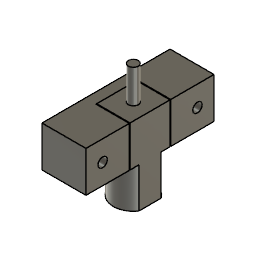
DC Motor (Autodesk Fusion 360 design; units mm, degrees)
Autodesk Fusion 360 part; units mm, degrees
sketch "Çizim1" plane through (0, 0, 0) normal (0, 0, 1) x (1, 0, 0)
  line L0 (5, 6) -> (-5, 6)
  line L1 (-5, 6) -> (-5, -6)
  line L2 (-5, -6) -> (5, -6)
  line L3 (5, -6) -> (5, 6)
  line L4 (5, 6) -> (-5, -6) construction
  line L5 (-5, 6) -> (5, -6) construction
  dimension "d1" = 10
  dimension "d2" = 12
  constraint horizontal L0
  constraint perpendicular L0 L1
  constraint parallel L0 L2
  constraint parallel L1 L3
  constraint coincident L4 origin
  constraint coincident L5 origin
  measures "d1" distance of L1.end L2.end
  measures "d2" distance of L0.end L1.end
extrude "Ekstrüzyon1" add sketch "Çizim1" along normal blind 24.2 makes body 1
sketch "Çizim2" plane through (0, 0, 24.2) normal (0, 0, 1) x (-1, 0, 0)
  line L0 (-5, 6) -> (-5, -6)
  line L1 (-5, -6) -> (5, -6)
  line L2 (5, -6) -> (5, 6)
  line L3 (5, 6) -> (-5, 6)
  circle A0 centre (0, 0) radius 1.5
  dimension "d5" = 3
  constraint coincident A0.centre origin
  measures "d5" diameter of A0
extrude "Ekstrüzyon2" add sketch "Çizim2" along normal blind 10 contours A0 bodies 1
sketch "Çizim3" plane through (0, 0, 0) normal (0, 0, -1) x (1, 0, 0)
  line L0 (5, -6) -> (5, 6)
  line L1 (5, 6) -> (-5, 6)
  line L2 (-5, 6) -> (-5, -6)
  line L3 (-5, -6) -> (5, -6)
  circle A0 centre (0, 0) radius 2.5
  dimension "d8" = 5
  constraint coincident A0.centre origin
  measures "d8" diameter of A0
extrude "Ekstrüzyon3" add sketch "Çizim3" along normal blind 1 contours A0 bodies 1
sketch "Çizim4" plane through (0, 0, 0) normal (0, 0, -1) x (1, 0, 0)
  circle A0 centre (0, 0) radius 2.5
  line L0 (5, -6) -> (5, 6)
  line L1 (5, 6) -> (-5, 6)
  line L2 (-5, 6) -> (-5, -6)
  line L3 (-5, -6) -> (5, -6)
  circle A1 centre (0, 0) radius 6
  dimension "d11" = 12
  constraint coincident A0.centre A1.centre
  measures "d11" diameter of A1
extrude "Ekstrüzyon4" cut sketch "Çizim4" against normal blind 12 contours L0 L3 A1 | L2 L3 A1 | L0 L1 A1 | L1 L2 A1 bodies 1
sketch "Çizim5" plane through (-5, 0, 0) normal (-1, 0, 0) x (0, -1, 0)
  line L0 (-3.3166, 12) -> (-3.3166, 0)
  line L1 (-3.3166, 0) -> (3.3166, 0)
  line L2 (3.3166, 0) -> (3.3166, 12)
  line L3 (3.3166, 12) -> (6, 12)
  line L4 (6, 12) -> (6, 24.2)
  line L5 (6, 24.2) -> (-6, 24.2)
  line L6 (-6, 24.2) -> (-6, 12)
  line L7 (-6, 12) -> (-3.3166, 12)
  line L8 (-6, 24.2) -> (6, 24.2)
  line L9 (6, 24.2) -> (6, 12)
  line L10 (6, 12) -> (-6, 12)
  line L11 (-6, 12) -> (-6, 24.2)
  line L12 (-6, 24.2) -> (-9.2, 24.2)
  line L13 (-9.2, 24.2) -> (-9.2, 12)
  line L14 (-9.2, 12) -> (-6, 12)
  line L15 (-6, 12) -> (-6, 24.2)
  line L16 (6, 24.2) -> (9.2, 24.2)
  line L17 (9.2, 24.2) -> (9.2, 12)
  line L18 (9.2, 12) -> (6, 12)
  line L19 (6, 12) -> (6, 24.2)
  dimension "d14" = 3.2
  dimension "d15" = 3.2
  constraint horizontal L8
  constraint vertical L9
  constraint horizontal L10
  constraint vertical L11
  constraint coincident L3.end L4.start
  constraint coincident L5.end L6.start
  constraint horizontal L12
  constraint vertical L13
  constraint horizontal L14
  constraint vertical L15
  constraint horizontal L16
  constraint vertical L17
  constraint horizontal L18
  constraint vertical L19
  constraint coincident L4.end L5.start
  constraint coincident L6.end L7.start
  measures "d14" distance of L13 L15
  measures "d15" distance of L9 L17
extrude "Ekstrüzyon5" add sketch "Çizim5" along normal blind 3.2 separate body contours L3 L4 L5 L6 L7 L8 L9 L10 L11 L15 L19 | L6 L11 L12 L13 L14 L15 | L4 L9 L16 L17 L18 L19 makes body 2
sketch "Çizim6" plane through (-5, 0, 0) normal (1, 0, 0) x (0, 1, 0)
  line L0 (9.2, 24.2) -> (-9.2, 24.2)
  line L1 (-9.2, 24.2) -> (-9.2, 12)
  line L2 (-9.2, 12) -> (9.2, 12)
  line L3 (9.2, 12) -> (9.2, 24.2)
  line L4 (-9.2, 24.2) -> (-6.2, 24.2)
  line L5 (-6.2, 24.2) -> (-6.2, 12)
  line L6 (-6.2, 12) -> (-9.2, 12)
  line L7 (-9.2, 12) -> (-9.2, 24.2)
  line L8 (9.2, 24.2) -> (6.2, 24.2)
  line L9 (6.2, 24.2) -> (6.2, 12)
  line L10 (6.2, 12) -> (9.2, 12)
  line L11 (9.2, 12) -> (9.2, 24.2)
  dimension "d18" = 3
  dimension "d19" = 3
  constraint horizontal L4
  constraint vertical L5
  constraint horizontal L6
  constraint vertical L7
  constraint coincident L0.end L1.start
  constraint horizontal L8
  constraint vertical L9
  constraint horizontal L10
  constraint vertical L11
  constraint coincident L0.start L3.end
  measures "d18" distance of L0.end L4.end
  measures "d19" distance of L0.start L8.end
extrude "Ekstrüzyon6" add sketch "Çizim6" along normal blind 10 contours L0 L2 L3 L8 L9 L10 L11 | L0 L1 L2 L4 L5 L6 L7 bodies 2
sketch "Çizim7" plane through (0, -9.2, 0) normal (0, -1, 0) x (1, 0, 0)
  line L0 (5, 24.2) -> (-8.2, 24.2)
  line L1 (-8.2, 24.2) -> (-8.2, 12)
  line L2 (-8.2, 12) -> (5, 12)
  line L3 (5, 12) -> (5, 24.2)
  line L4 (5, 24.2) -> (0, 24.2)
  line L5 (0, 24.2) -> (0, 12)
  line L6 (0, 12) -> (5, 12)
  line L7 (5, 12) -> (5, 24.2)
  dimension "d22" = 5
  constraint horizontal L4
  constraint vertical L5
  constraint horizontal L6
  constraint vertical L7
  constraint coincident L2 L5.end
  constraint coincident L0.start L3.end
  measures "d22" distance of L0.start L4.end
extrude "Ekstrüzyon7" add sketch "Çizim7" along normal blind 10 contours L0 L2 L3 L4 L5 L6 L7 bodies 2
sketch "Çizim8" plane through (0, 9.2, 0) normal (0, 1, 0) x (-1, 0, 0)
  line L0 (-5, 12) -> (8.2, 12)
  line L1 (8.2, 12) -> (8.2, 24.2)
  line L2 (8.2, 24.2) -> (-5, 24.2)
  line L3 (-5, 24.2) -> (-5, 12)
  line L4 (-5, 24.2) -> (0, 24.2)
  line L5 (0, 24.2) -> (0, 12)
  line L6 (0, 12) -> (-5, 12)
  line L7 (-5, 12) -> (-5, 24.2)
  dimension "d25" = 5
  dimension "d26" = 12.2
  constraint horizontal L4
  constraint vertical L5
  constraint horizontal L6
  constraint vertical L7
  constraint coincident L2.end L3.start
  measures "d25" distance of L2.end L4.end
  measures "d26" distance of L2.end L0.start
extrude "Ekstrüzyon8" add sketch "Çizim8" along normal blind 10 contours L0 L2 L3 L4 L5 L6 L7 bodies 2
sketch "Çizim9" plane through (0, 0, 0) normal (-1, 0, 0) x (0, -1, 0)
  line L0 (9.2, 24.2) -> (9.2, 12)
  line L1 (9.2, 12) -> (19.2, 12)
  line L2 (19.2, 12) -> (19.2, 24.2)
  line L3 (19.2, 24.2) -> (9.2, 24.2)
  line L4 (19.2, 18.1) -> (9.2, 18.1)
  line L5 (14.2, 12) -> (14.2, 18.1)
  circle A0 centre (14.2, 18.1) radius 1.4
  dimension "d29" = 2.8
  constraint midpoint L2 L4.start
  constraint midpoint L0 L4.end
  constraint midpoint L1 L5.start
  constraint midpoint L4 L5.end
  constraint coincident L5.end A0.centre
  measures "d29" diameter of A0
extrude "Ekstrüzyon9" cut sketch "Çizim9" against normal blind 5 contours L4 A0 | L4 L5 A0 | L4 L5 A0 bodies 2
mirror "Ayna1" about plane through (0, 0, 0) normal (0, 1, 0) of "Ekstrüzyon9"
extrude "Ekstrüzyon10" add 2 faces at (0, -14.2349, 22.632) (0, 14.1651, 13.568) along direction (-1, 0, 0) blind 8.2 on bodies 2 bodies 2
equation "d18 = 3.2 mm - 0.2 mm"
